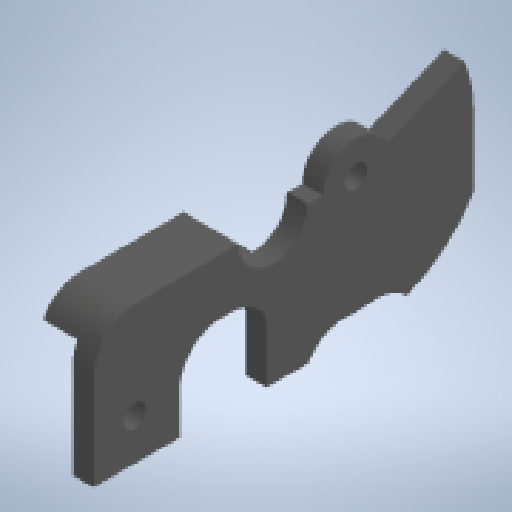
# Autodesk Inventor part: toe_springjoint_cover_under_left
Saved by Autodesk Inventor 2024.1 (Build 281209000, 209)
## iProperties
Created: 2024-02-25
Part Number: toe_springjoint_cover_under_left
Material: 一般
Document SubType Name: Modeling
Designer: hibik
Density: 1 g/cm^3
Appearance: 既定
Author: hibik
Autodesk Inventor part; units mm, degrees
ref_plane "YZ Plane" through (0, 0, 0) normal (1, 0, 0) x (0, 1, 0)
ref_plane "XZ Plane" through (0, 0, 0) normal (0, 1, 0) x (-1, 0, 0)
ref_plane "XY Plane" through (0, 0, 0) normal (0, 0, 1) x (1, 0, 0)
sketch "スケッチ1" plane through (0, 0, 0) normal (1, 0, 0) x (0, 1, 0)
  circle A0 centre (0, 0) radius 6 construction
  circle A1 centre (6, 0) radius 0.8
  line L0 (-14, 0) -> (14, 0) projected
  circle A2 centre (4.2426, 4.2426) radius 0.8
  circle A3 centre (0, 6) radius 0.8
  circle A4 centre (-4.2426, 4.2426) radius 0.8
  circle A5 centre (-6, 0) radius 0.8
  circle A6 centre (-4.2426, -4.2426) radius 0.8
  circle A7 centre (0, -6) radius 0.8
  circle A8 centre (4.2426, -4.2426) radius 0.8
  circle A9 centre (0, 0) radius 2.4
  line L1 (0, 0) -> (0, 6)
  line L2 (0, 0) -> (2.2961, -5.5433)
  circle A10 centre (0, 0) radius 10
  line L3 (2.2961, -5.5433) -> (3.8268, -9.2388)
  line L4 (0, -9.2388) -> (-10, -9.2388)
  line L5 (-10, -9.2388) -> (-10, 20)
  line L6 (-10, 20) -> (0, 20)
  line L7 (0, 20) -> (0, -9.2388)
  line L8 (0, -6) -> (4.2426, -4.2426) construction
  line L9 (0, -9.2388) -> (3.8268, -9.2388)
  circle A11 centre (0, 6) radius 2.5
  point P0 (0, 5.2)
  point P1 (0, 6.8)
  point P2 (-10, 0)
  point P3 (2.1213, -5.1213)
  point P4 (0, 2.4)
  point P5 (0.9184, -2.2173)
  point P6 (0, 8.5)
  point P7 (0, 10)
  point P8 (0, 3.5)
  point P9 (-3.8268, -9.2388)
  point P10 (0, -6.8)
  point P11 (0, -5.2)
  point P12 (0, -2.4)
  dimension "d1" = 12
  dimension "d2" = 1.6
  dimension "d5" = 360
  dimension "d7" = 4.8
  dimension "d8" = 4
  dimension "d21" = 5
  dimension "d23" = 20
  constraints: 18 end point, 11 centre point, 6 point on line, 5 coincident, 3 point on circle, 2 horizontal, 2 parallel, 1 midpoint, 1 perpendicular, 1 vertical, 20 other
  measures "d1" diameter of A0
  measures "d2" diameter of A1
  measures "d7" diameter of A9
  measures "d21" diameter of A11
  measures "d23" distance from line of L6 point (0, 0)
extrude "押し出し1" add sketch "スケッチ1" along normal blind 1.5 contours A9 L2 L0 | L0 L1 A9 | L9 L7 A7 A9 L2 L3 | L7 A11 L1 A9 L0 A5 A10 | A10 L5 L6 L7 | L7 A9 L0 | L0 A9 L1 | L2 A9 L7 | L4 L5 A10 | A10 L0 A5 A9 L7 A7 L4 | L7 A7 | A7 L7 | A5 L0 | L0 A5 | A4 | A6
sketch "スケッチ6" plane through (0, 0, 0) normal (-1, 0, 0) x (0, 0, 1)
  line L0 (12.7468, -7) -> (12.7468, -10) projected
  line L1 (19, -10) -> (12.7468, -10) projected
  line L2 (19, -10) -> (19, -3) projected
  arc A0 (19, -3) -> (16, 0) centre (16, -3) ccw projected
  line L3 (8.5, 0) -> (16, 0) projected
  arc A1 (3.9844, 1.4789) -> (8.5, 0) centre (6, 0) ccw projected
  arc A2 (3.9844, 1.4789) -> (-3.9265, 1.6264) centre (0, 0) ccw projected
  line L4 (-7.853, 3.2528) -> (-3.9265, 1.6264) projected
  arc A3 (-7.853, 3.2528) -> (-8.5, 0) centre (0, 0) ccw projected
  line L5 (-8.5, 0) -> (-8.5, -5.2678) projected
  arc A4 (-8.5, -5.2678) -> (-3.6504, -9.3099) centre (0, 0) ccw projected
  arc A5 (-1.1087, -8.4274) -> (-3.6504, -9.3099) centre (-1.5, -11.4018) ccw projected
  arc A6 (-1.1087, -8.4274) -> (0.6267, -8.4769) centre (0, 0) ccw projected
  arc A7 (3.446, -9.9687) -> (0.6267, -8.4769) centre (0.848, -11.4687) ccw projected
  line L6 (3.446, -9.9687) -> (3.4641, -10) projected
  line L7 (6.4797, -10) -> (3.4641, -10) projected
  line L8 (6.4797, -10) -> (6.4797, -6.5597) projected
  arc A8 (6.7439, -5.1739) -> (6.4797, -6.5597) centre (9.4761, -6.413) ccw projected
  arc A9 (9.1241, -4) -> (6.7439, -5.1739) centre (9.1241, -7) ccw projected
  line L9 (9.1241, -4) -> (9.7468, -4) projected
  arc A10 (12.7468, -7) -> (9.7468, -4) centre (9.7468, -7) ccw projected
  circle A11 centre (17, -3.5) radius 0.8 projected
  circle A12 centre (-6, 0) radius 0.8 projected
  circle A13 centre (-4.2426, -4.2426) radius 0.8 projected
  circle A14 centre (4.2426, -4.2426) radius 0.8 projected
  circle A15 centre (0, -6) radius 0.8 projected
  arc A16 (2.4, 0) -> (-2.2173, 0.9184) centre (0, 0) ccw projected
  line L10 (-9.2388, 3.8268) -> (-2.2173, 0.9184) projected
  line L11 (-9.2388, -10) -> (-9.2388, 3.8268) projected
  line L12 (20, -10) -> (-9.2388, -10) projected
  line L13 (20, 0) -> (20, -10) projected
  line L14 (8.5, 0) -> (20, 0) projected
  arc A17 (3.5, 0) -> (8.5, 0) centre (6, 0) ccw projected
  line L15 (2.4, 0) -> (3.5, 0) projected
  circle A18 centre (16, -7) radius 0.8 projected
  circle A19 centre (0, 0) radius 0.8 projected
  point P0 (16, 0)
extrude "押し出し5" cut sketch "スケッチ6" against normal through all contours L0 L12 L8 A8 A9 L9 A10 | L2 A0 L14 L13 L12 | L12 L11 L10 A3 L5 A4 A5 A6 A7 L6
sketch "スケッチ7" plane through (0, 0, 0) normal (-1, 0, 0) x (0, 0, 1)
  line L0 (14.5, -3.5) -> (6.6298, -3.5) projected
  arc A0 (-7.853, 3.2528) -> (-8.5, 0) centre (0, 0) ccw projected
  line L1 (-8.5, 0) -> (-8.5, -5.2678) projected
  arc A1 (-8.5, -5.2678) -> (-3.6504, -9.3099) centre (0, 0) ccw projected
  arc A2 (-1.1087, -8.4274) -> (-3.6504, -9.3099) centre (-1.5, -11.4018) ccw projected
  arc A3 (-1.1087, -8.4274) -> (0.6267, -8.4769) centre (0, 0) ccw projected
  arc A4 (3.446, -9.9687) -> (0.6267, -8.4769) centre (0.848, -11.4687) ccw projected
  line L2 (3.446, -9.9687) -> (3.4641, -10) projected
  line L3 (6.4797, -10) -> (3.4641, -10) projected
  line L4 (6.4797, -10) -> (6.4797, -6.5597) projected
  arc A5 (6.7439, -5.1739) -> (6.4797, -6.5597) centre (9.4761, -6.413) ccw projected
  arc A6 (9.1241, -4) -> (6.7439, -5.1739) centre (9.1241, -7) ccw projected
  line L5 (9.1241, -4) -> (9.7468, -4) projected
  arc A7 (12.7468, -7) -> (9.7468, -4) centre (9.7468, -7) ccw projected
  line L6 (12.7468, -7) -> (12.7468, -10) projected
  line L7 (19, -10) -> (12.7468, -10) projected
  line L8 (19, -10) -> (19, -3) projected
  arc A8 (19, -3) -> (16, 0) centre (16, -3) ccw projected
  line L9 (8.5, 0) -> (16, 0) projected
  arc A9 (3.5, 0) -> (8.5, 0) centre (6, 0) ccw projected
  line L10 (2.4, 0) -> (3.5, 0) projected
  arc A10 (2.4, 0) -> (-2.2173, 0.9184) centre (0, 0) ccw projected
  line L11 (-7.853, 3.2528) -> (-2.2173, 0.9184) projected
  circle A11 centre (17, -3.5) radius 0.8 projected
  circle A12 centre (17, -3.5) radius 2.5
  line L12 (6.6298, -3.5) -> (0, -3.5)
  circle A13 centre (0, 0) radius 3.5
  line L13 (3.5, 0) -> (3.5, -3.5)
  line L14 (0, -3.5) -> (14.7087, -3.5)
  line L15 (14.7087, -3.5) -> (14.7087, -2.5)
  line L16 (14.7087, -2.5) -> (0, -2.5)
  line L17 (0, -2.5) -> (0, -3.5)
  point P0 (18.677, -1.6459)
  point P1 (6, -2.5)
  dimension "d31" = 5
  dimension "d34" = 1
  constraints: 12 end point, 3 horizontal, 2 coincident, 2 parallel, 2 perpendicular, 1 collinear, 1 point on line, 1 tangent, 1 vertical, 1 vertical alignment, 5 other
  measures "d34" distance between parallel lines of L16 L0
extrude "押し出し6" add sketch "スケッチ7" along normal blind 2.5 contours L16 A9 L9 A8 A12
sketch "スケッチ8" plane through (1.5, 0, 0) normal (1, 0, 0) x (0, 0, -1)
  circle A0 centre (-16, -7) radius 0.8
  line L0 (-19, -10) -> (-12.7468, -10) projected
  line L1 (-19, -3) -> (-19, -10) projected
  circle A1 centre (0, 0) radius 0.8
  dimension "d35" = 1.6
  dimension "d36" = 3
  dimension "d37" = 3
  dimension "d40" = 1.6
  constraints: 2 centre point, 1 coincident
  measures "d35" diameter of A0
  measures "d36" distance from line of L0 A0.centre
  measures "d37" distance from line of L1 A0.centre
  measures "d40" diameter of A1
extrude "押し出し7" cut sketch "スケッチ8" against normal through all
